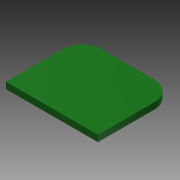
# Autodesk Inventor part: Platine encodeur
Saved by Autodesk Inventor 2014 SP2 (Build 180246200, 246)
## iProperties
Created: 2015-03-17
Part Number: Platine encodeur
Material: Verre
Document SubType Name: Modeling
Designer: sd
Density: 2.18 g/cm^3
Appearance: Clair
Mass: 0.194212 g
Surface Area: 2.5664 cm^2
Volume: 0.089088 cm^3
Author: sd
Autodesk Inventor part; units mm, degrees
ref_plane "YZ Plane" through (0, 0, 0) normal (1, 0, 0) x (0, 1, 0)
ref_plane "XZ Plane" through (0, 0, 0) normal (0, 1, 0) x (-1, 0, 0)
ref_plane "XY Plane" through (0, 0, 0) normal (0, 0, 1) x (1, 0, 0)
sketch "Esquisse1" plane through (0, 0, 0) normal (0, 0, 1) x (1, 0, 0)
  line L0 (-5.8, -4.8) -> (5.8, -4.8)
  line L1 (5.8, -4.8) -> (5.8, 4.8)
  line L2 (5.8, 4.8) -> (-5.8, 4.8)
  line L3 (-5.8, 4.8) -> (-5.8, -4.8)
  point P0 (0, 0)
  dimension "d0" = 11.6
  dimension "d1" = 9.6
  dimension "d2" = 4.8
  dimension "d3" = 5.8
  constraints: 8 end point, 2 parallel, 1 horizontal, 1 perpendicular
  measures "d0" distance of L1.end L2.end
  measures "d1" distance of L2.end L0.start
  measures "d2" vertical distance of point (0, 0) L2.end
  measures "d3" horizontal distance of point (0, 0) L2.end
extrude "Extrusion1" add sketch "Esquisse1" along normal blind 0.8
fillet "Congé1" radius 2.5 2 edges at (-5.8, 4.8, 0.4) (5.8, 4.8, 0.4)
equation "\"d2\" = 0.5 * d1"
equation "\"d3\" = 0.5 * d0"
